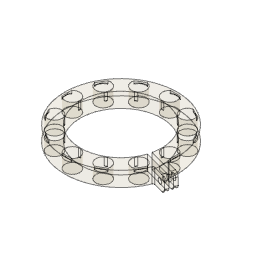
clamp-rev3 v4 (Autodesk Fusion 360 design; units mm, degrees)
Autodesk Fusion 360 part; units mm, degrees
note: some values were not read from the file. Set by a fixed rule: which face or edge a step refers to.
sketch "Sketch1" plane through (0, 0, 9.525) normal (0, 0, 1) x (-1, 0, 0) in component "magnet holder"
  arc A0 (0, -47.625) -> (-95.25, -47.625) centre (-47.625, -47.625) ccw
  line L0 (-95.25, -47.625) -> (-95.25, -130.175)
  arc A1 (-95.25, -130.175) -> (0, -130.175) centre (-47.625, -130.175) ccw
  line L1 (0, -130.175) -> (0, -47.625)
  circle A2 centre (-47.625, -130.175) radius 35.306
  circle A3 centre (-47.625, -130.175) radius 47.625
  circle A4 centre (-47.625, -130.175) radius 35.306
  circle A5 centre (-47.625, -41.275) radius 39.37
  circle A6 centre (-18.3045, -159.4955) radius 2.159
  circle A7 centre (-76.9455, -159.4955) radius 2.159
  circle A8 centre (-18.3045, -100.8545) radius 2.159
  circle A9 centre (-76.9455, -100.8545) radius 2.159
  dimension "d96_1" = 4.318
  dimension "d97_1" = 4.318
  dimension "d98_1" = 4.318
  dimension "d99_1" = 4.318
  constraint concentric A1 A3
  constraint concentric A3 A4
  measures "d96_1" diameter of A6
  measures "d97_1" diameter of A7
  measures "d98_1" diameter of A8
  measures "d99_1" diameter of A9
extrude "Extrude1" add sketch "Sketch1" along normal blind 5.588 contours A1 A3 in component "magnet holder"
sketch "Sketch2" plane through (0, 0, 9.525) normal (0, 0, -1) x (1, 0, 0) in component "magnet holder"
  circle A0 centre (47.625, -130.175) radius 35.306
  circle A1 centre (47.625, -130.175) radius 47.625
  circle A2 centre (47.625, -130.175) radius 41.4655 construction
  circle A3 centre (47.625, -88.7095) radius 6
  circle A4 centre (26.8922, -94.2648) radius 6
  circle A5 centre (11.7148, -109.4422) radius 6
  circle A6 centre (6.1595, -130.175) radius 6
  circle A7 centre (11.7148, -150.9077) radius 6
  circle A8 centre (26.8922, -166.0852) radius 6
  circle A9 centre (47.625, -171.6405) radius 6
  circle A10 centre (68.3577, -166.0852) radius 6
  circle A11 centre (83.5352, -150.9078) radius 6
  circle A12 centre (89.0905, -130.175) radius 6
  circle A13 centre (83.5352, -109.4423) radius 6
  circle A14 centre (68.3578, -94.2648) radius 6
  circle A15 centre (76.9455, -100.8545) radius 2.159
  circle A16 centre (18.3045, -100.8545) radius 2.159
  circle A17 centre (18.3045, -159.4955) radius 2.159
  circle A18 centre (76.9455, -159.4955) radius 2.159
  dimension "d91_1" = 12
  dimension "d93_1" = 360
  constraint concentric A0 A2
  constraint coincident A2 A3.centre
  measures "d91_1" diameter of A3
extrude "Extrude2" cut sketch "Sketch2" against normal blind 4.0005 contours A3 | A4 | A5 | A6 | A7 | A8 | A9 | A10 | A11 | A12 | A13 | A14 in component "magnet holder"
sketch "Sketch1 (2)" plane through (0, 0, 15.875) normal (0, 0, 1) x (-1, 0, 0) in component "magnet spacer"
  circle A0 centre (-76.9455, -100.8545) radius 1.651
  circle A1 centre (-18.3045, -100.8545) radius 1.651
  circle A2 centre (-18.3045, -159.4955) radius 1.651
  circle A3 centre (-76.9455, -159.4955) radius 1.651
  circle A4 centre (-47.625, -130.175) radius 35.306
  circle A5 centre (-47.625, -130.175) radius 47.625
  circle A6 centre (-47.625, -130.175) radius 47.625
  circle A7 centre (-18.3045, -159.4955) radius 1.651
  circle A8 centre (-76.9455, -159.4955) radius 1.651
  circle A9 centre (-76.9455, -100.8545) radius 1.651
  circle A10 centre (-18.3045, -100.8545) radius 1.651
  constraint concentric A4 A6
  constraint concentric A2 A7
  constraint concentric A3 A8
  constraint concentric A0 A9
  constraint concentric A1 A10
sketch "Sketch1 (3)" plane through (0, 0, 16.6622) normal (0, 0, 1) x (-1, 0, 0)
  circle A0 centre (-11.7148, -109.4423) radius 6
  circle A1 centre (-83.5352, -150.9077) radius 6
  circle A2 centre (-11.7148, -150.9078) radius 6
  circle A3 centre (-6.1595, -130.175) radius 6
  circle A4 centre (-89.0905, -130.175) radius 6
  circle A5 centre (-26.8922, -94.2648) radius 6
  circle A6 centre (-68.3577, -94.2648) radius 6
  circle A7 centre (-68.3577, -166.0852) radius 6
  circle A8 centre (-26.8922, -166.0852) radius 6
  circle A9 centre (-47.625, -171.6405) radius 6
  circle A10 centre (-83.5352, -109.4422) radius 6
  circle A11 centre (-47.625, -88.7095) radius 6
  circle A12 centre (-76.9455, -159.4955) radius 2.159
  circle A13 centre (-47.625, -130.175) radius 35.306
  circle A14 centre (-76.9455, -100.8545) radius 2.159
  circle A15 centre (-18.3045, -159.4955) radius 2.159
  circle A16 centre (-18.3045, -100.8545) radius 2.159
  circle A17 centre (-47.625, -130.175) radius 47.625
  line L0 (-53.625, -88.7095) -> (-53.625, -82.8628)
  line L1 (-41.6392, -89.1226) -> (-41.6392, -82.7277)
  line L2 (-73.5539, -97.2648) -> (-76.4772, -92.2015)
  line L3 (-62.9674, -91.6297) -> (-66.1648, -86.0915)
  line L4 (-86.5352, -114.6384) -> (-91.5985, -111.7151)
  line L5 (-80.1845, -104.465) -> (-85.7227, -101.2675)
  line L6 (-89.0905, -136.175) -> (-94.9372, -136.175)
  line L7 (-88.6774, -124.1892) -> (-95.0723, -124.1892)
  line L8 (-80.5352, -156.1039) -> (-85.5985, -159.0272)
  line L9 (-86.1703, -145.5174) -> (-91.7085, -148.7148)
  line L10 (-63.1616, -169.0852) -> (-66.0849, -174.1485)
  line L11 (-73.335, -162.7345) -> (-76.5325, -168.2727)
  line L12 (-41.625, -171.6405) -> (-41.625, -177.4872)
  line L13 (-53.6108, -171.2274) -> (-53.6108, -177.6223)
  line L14 (-21.6961, -163.0852) -> (-18.7728, -168.1485)
  line L15 (-32.2826, -168.7203) -> (-29.0852, -174.2585)
  line L16 (-8.7148, -145.7116) -> (-3.6515, -148.6349)
  line L17 (-15.0655, -155.885) -> (-9.5273, -159.0825)
  line L18 (-6.1595, -124.175) -> (-0.3128, -124.175)
  line L19 (-6.5726, -136.1608) -> (-0.1777, -136.1608)
  line L20 (-14.7148, -104.2461) -> (-9.6515, -101.3228)
  line L21 (-9.0797, -114.8326) -> (-3.5415, -111.6352)
  line L22 (-32.0884, -91.2648) -> (-29.1651, -86.2015)
  line L23 (-21.915, -97.6155) -> (-18.7175, -92.0773)
  point P0 (-53.625, -88.7095)
  dimension "d2" = 360
  constraint coincident P0 L0.start
  constraint vertical L0
  constraint coincident A11 L1.start
  constraint vertical L1
sketch "Sketch2 (2)" plane through (0, 0, 16.6622) normal (0, 0, 1) x (-1, 0, 0)
  circle A0 centre (-76.9455, -159.4955) radius 2.159
  circle A1 centre (-47.625, -130.175) radius 35.306
  circle A2 centre (-76.9455, -100.8545) radius 2.159
  circle A3 centre (-18.3045, -159.4955) radius 2.159
  circle A4 centre (-18.3045, -100.8545) radius 2.159
  circle A5 centre (-47.625, -130.175) radius 47.625
  circle A6 centre (-47.625, -130.175) radius 35.306
  circle A7 centre (-11.7148, -109.4423) radius 6
  circle A8 centre (-83.5352, -150.9077) radius 6
  circle A9 centre (-11.7148, -150.9078) radius 6
  circle A10 centre (-6.1595, -130.175) radius 6
  circle A11 centre (-89.0905, -130.175) radius 6
  circle A12 centre (-26.8922, -94.2648) radius 6
  circle A13 centre (-68.3577, -94.2648) radius 6
  circle A14 centre (-68.3577, -166.0852) radius 6
  circle A15 centre (-26.8922, -166.0852) radius 6
  circle A16 centre (-47.625, -171.6405) radius 6
  circle A17 centre (-83.5352, -109.4422) radius 6
  circle A18 centre (-47.625, -88.7095) radius 6
  circle A19 centre (-47.625, -130.175) radius 47.625
  dimension "d61" = 70.612
  constraint concentric A5 A6
  measures "d61" diameter of A6
extrude "Extrude4" add sketch "Sketch2 (2)" along normal blind 7.112 contours A5 A19 | A7 | A8 | A9 | A10 | A11 | A12 | A13 | A14 | A15 | A16 | A17 | A18 sketch seen with x (-1, 0, 0) y (0, 1, 0) z (0, 0, -1) at (95.25, 0, 26.1872) in component "magnet holder"
extrude "Extrude5" cut 12 faces at (66.4689, 94.5562, 9.525) (49.4935, 89.8687, 9.525) (25.3169, 97.0824, 9.525) (10.5654, 105.7158, 9.525) (6.8902, 133.2158, 9.525) (10.9841, 149.046, 9.525) (26.1616, 167.9469, 9.525) (50.8883, 170.7727, 9.525) (67.6271, 167.9469, 9.525) (80.2719, 151.7755, 9.525) (85.5579, 131.1725, 9.525) (81.9599, 112.2599, 9.525) along direction (0, 0, -1) through all in component "magnet holder"
extrude "Extrude6" cut 12 faces at (81.9802, 105.2788, 13.5255) (89.6447, 133.5821, 13.5255) (80.8432, 151.7755, 13.5255) (67.6271, 167.9469, 13.5255) (50.8883, 170.7727, 13.5255) (26.1616, 167.9469, 13.5255) (10.9841, 149.046, 13.5255) (6.6045, 131.9486, 13.5255) (10.1395, 112.2599, 13.5255) (28.8699, 95.1458, 13.5255) (49.4935, 89.8687, 13.5255) (67.3578, 90.2795, 13.5255) along direction (0, 0, 1) blind 0.5842 in component "magnet holder"
sketch "Sketch3" plane through (0, 0, 23.7742) normal (0, 0, 1) x (-1, 0, 0)
  circle A0 centre (-6.1595, -130.175) radius 6
  circle A1 centre (-26.8922, -166.0852) radius 6
  circle A2 centre (-68.3577, -166.0852) radius 6
  circle A3 centre (-89.0905, -130.175) radius 6
  circle A4 centre (-68.3577, -94.2648) radius 6
  circle A5 centre (-26.8922, -94.2648) radius 6
  circle A6 centre (-47.625, -88.7095) radius 6
  circle A7 centre (-83.5352, -109.4422) radius 6
  circle A8 centre (-83.5352, -150.9077) radius 6
  circle A9 centre (-47.625, -171.6405) radius 6
  circle A10 centre (-11.7148, -150.9078) radius 6
  circle A11 centre (-11.7148, -109.4423) radius 6
  circle A12 centre (-18.3045, -159.4955) radius 2.159
  circle A13 centre (-18.3045, -100.8545) radius 2.159
  circle A14 centre (-76.9455, -100.8545) radius 2.159
  circle A15 centre (-76.9455, -159.4955) radius 2.159
  circle A16 centre (-47.625, -130.175) radius 35.306
  circle A17 centre (-47.625, -130.175) radius 47.625
  circle A18 centre (-47.625, -130.175) radius 47.875
  dimension "d10" = 0.25
  constraint concentric A16 A18
  measures "d10" distance of A17 A18
extrude "Extrude7" add sketch "Sketch3" against normal up to surface (12.7 mm away) contours A18 sketch seen with x (-1, 0, 0) y (0, 1, 0) z (0, 0, -1) at (95.25, 0, 26.1872) in component "magnet holder"
move_face "OffsetFaces1" offset -0.254 3 faces at (42.0961, 169.3099, 4.7837) (42.0961, 173.9711, 12.192) (42.0961, 173.9711, 13.915) in component "magnet holder"
move_face "OffsetFaces2" offset -0.254 3 faces at (73.8866, 163.7546, 4.7837) (63.0884, 163.2157, 12.192) (63.238, 162.9566, 13.915) in component "magnet holder"
move_face "OffsetFaces3" offset -0.254 3 faces at (89.064, 148.5771, 4.7837) (78.0063, 153.2384, 12.192) (77.897, 152.9599, 13.7202) in component "magnet holder"
move_face "OffsetFaces4" offset -0.254 3 faces at (83.5616, 132.5056, 7.1543) (83.5616, 132.5056, 12.192) (83.4523, 132.2271, 13.7202) in component "magnet holder"
move_face "OffsetFaces5" offset -0.254 3 faces at (89.5054, 108.8448, 4.7837) (77.565, 110.0397, 12.192) (77.5426, 109.7413, 13.7202) in component "magnet holder"
move_face "OffsetFaces6" offset -0.254 3 faces at (74.3279, 93.6674, 4.7837) (62.3876, 94.8622, 12.192) (62.3652, 94.5639, 13.7202) in component "magnet holder"
move_face "OffsetFaces7" offset -0.254 3 faces at (53.5952, 88.1121, 4.7837) (41.6548, 89.3069, 12.192) (41.6325, 89.0086, 13.7202) in component "magnet holder"
move_face "OffsetFaces8" offset -0.254 3 faces at (32.8624, 93.6674, 4.7837) (32.8624, 94.8622, 12.192) (32.8624, 94.8622, 13.7202) in component "magnet holder"
move_face "OffsetFaces9" offset -0.254 3 faces at (17.685, 108.8448, 4.7837) (17.685, 110.0397, 12.192) (17.685, 110.0397, 13.7202) in component "magnet holder"
move_face "OffsetFaces10" offset -0.254 3 faces at (0.6306, 132.5056, 7.1543) (0.6306, 132.5056, 12.192) (0.6306, 132.5056, 13.915) in component "magnet holder"
move_face "OffsetFaces11" offset -0.254 3 faces at (6.186, 148.5771, 4.7837) (6.186, 153.2384, 12.192) (6.186, 153.2384, 13.915) in component "magnet holder"
move_face "OffsetFaces12" offset -0.254 3 faces at (32.4211, 163.7546, 4.7837) (32.012, 162.9566, 12.192) (32.012, 162.9566, 13.915) in component "magnet holder"
sketch "Sketch4" plane through (0, 0, 23.7742) normal (0, 0, 1) x (-1, 0, 0)
  circle A0 centre (-47.625, -130.175) radius 47.875
  circle A1 centre (-18.3045, -159.4955) radius 2.159
  circle A2 centre (-18.3045, -100.8545) radius 2.159
  circle A3 centre (-76.9455, -100.8545) radius 2.159
  circle A4 centre (-76.9455, -159.4955) radius 2.159
  arc A5 (-66.1364, -160.239) -> (-64.4055, -161.2383) centre (-68.3577, -166.0852) ccw
  arc A6 (-77.689, -148.6864) -> (-66.1364, -160.239) centre (-47.625, -130.175) ccw
  arc A7 (-78.6883, -146.9555) -> (-77.689, -148.6864) centre (-83.5352, -150.9077) ccw
  arc A8 (-82.9169, -131.1743) -> (-78.6883, -146.9555) centre (-47.625, -130.175) ccw
  arc A9 (-82.9169, -129.1757) -> (-82.9169, -131.1743) centre (-89.0905, -130.175) ccw
  arc A10 (-78.6883, -113.3945) -> (-82.9169, -129.1757) centre (-47.625, -130.175) ccw
  arc A11 (-77.689, -111.6636) -> (-78.6883, -113.3945) centre (-83.5352, -109.4422) ccw
  arc A12 (-66.1364, -100.111) -> (-77.689, -111.6636) centre (-47.625, -130.175) ccw
  arc A13 (-64.4055, -99.1117) -> (-66.1364, -100.111) centre (-68.3577, -94.2648) ccw
  arc A14 (-48.6243, -94.8831) -> (-64.4055, -99.1117) centre (-47.625, -130.175) ccw
  arc A15 (-46.6257, -94.8831) -> (-48.6243, -94.8831) centre (-47.625, -88.7095) ccw
  arc A16 (-30.8445, -99.1117) -> (-46.6257, -94.8831) centre (-47.625, -130.175) ccw
  arc A17 (-29.1136, -100.111) -> (-30.8445, -99.1117) centre (-26.8922, -94.2648) ccw
  arc A18 (-17.561, -111.6636) -> (-29.1136, -100.111) centre (-47.625, -130.175) ccw
  arc A19 (-16.5617, -113.3945) -> (-17.561, -111.6636) centre (-11.7148, -109.4423) ccw
  arc A20 (-12.3331, -129.1757) -> (-16.5617, -113.3945) centre (-47.625, -130.175) ccw
  arc A21 (-12.3331, -131.1743) -> (-12.3331, -129.1757) centre (-6.1595, -130.175) ccw
  arc A22 (-16.5617, -146.9555) -> (-12.3331, -131.1743) centre (-47.625, -130.175) ccw
  arc A23 (-17.561, -148.6864) -> (-16.5617, -146.9555) centre (-11.7148, -150.9078) ccw
  arc A24 (-29.1136, -160.239) -> (-17.561, -148.6864) centre (-47.625, -130.175) ccw
  arc A25 (-30.8445, -161.2383) -> (-29.1136, -160.239) centre (-26.8922, -166.0852) ccw
  arc A26 (-46.6257, -165.4669) -> (-30.8445, -161.2383) centre (-47.625, -130.175) ccw
  arc A27 (-48.6243, -165.4669) -> (-46.6257, -165.4669) centre (-47.625, -171.6405) ccw
  arc A28 (-64.4055, -161.2383) -> (-48.6243, -165.4669) centre (-47.625, -130.175) ccw
  circle A29 centre (-47.625, -130.175) radius 46.2875
  dimension "d25" = 1.5875
  constraint concentric A0 A29
  measures "d25" distance of A0 A29
extrude "Extrude8" add sketch "Sketch4" against normal blind 1.27 contours A0 | A5 A29 | A7 A29 | A27 A29 | A9 A29 | A25 A29 | A11 A29 | A23 A29 | A13 A29 | A21 A29 | A15 A29 | A19 A29 | A17 A29 sketch seen with x (-1, 0, 0) y (0, 1, 0) z (0, 0, -1) at (95.25, 0, 26.1872) in component "magnet holder"
fillet "Fillet1" radius 1.27 1 edges at (47.625, 177.8945, 3.683) in component "magnet holder"
fillet "Fillet2" radius 1.27 1 edges at (71.4848, 171.5013, 3.683) in component "magnet holder"
fillet "Fillet3" radius 1.27 1 edges at (88.9513, 154.0348, 3.683) in component "magnet holder"
fillet "Fillet4" radius 1.27 1 edges at (95.3445, 130.175, 3.683) in component "magnet holder"
fillet "Fillet5" radius 1.27 1 edges at (88.9513, 106.3153, 3.683) in component "magnet holder"
fillet "Fillet6" radius 1.27 1 edges at (71.4848, 88.8487, 3.683) in component "magnet holder"
fillet "Fillet7" radius 1.27 1 edges at (47.625, 82.4555, 3.683) in component "magnet holder"
fillet "Fillet8" radius 1.27 1 edges at (23.7652, 88.8487, 3.683) in component "magnet holder"
fillet "Fillet9" radius 1.27 1 edges at (6.2987, 106.3152, 3.683) in component "magnet holder"
fillet "Fillet10" radius 1.27 1 edges at (-0.0945, 130.175, 3.683) in component "magnet holder"
fillet "Fillet11" radius 1.27 1 edges at (6.2987, 154.0348, 3.683) in component "magnet holder"
fillet "Fillet12" radius 1.27 1 edges at (23.7652, 171.5013, 3.683) in component "magnet holder"
ref_plane "WorkPlane1" through (47.625, 130.175, 24.5362) normal (0.258819, 0.965926, 0) x (0, 0, -1)
ref_plane "WorkPlane2" through (93.8687, 117.784, 17.4242) normal (0.965926, -0.258819, 0) x (-0.258819, -0.965926, 0)
sketch "Sketch10" plane through (93.8687, 117.784, 17.4242) normal (0.965926, -0.258819, 0) x (-0.258819, -0.965926, 0)
  line L0 (-4.7625, -6.35) -> (4.7625, -6.35)
  line L1 (4.7625, -6.35) -> (4.7625, 6.35)
  line L2 (4.7625, 6.35) -> (-4.7625, 6.35)
  line L3 (-4.7625, 6.35) -> (-4.7625, -6.35)
  line L4 (-4.7625, -6.35) -> (4.7625, 6.35) construction
  line L5 (4.7625, -6.35) -> (-4.7625, 6.35) construction
  line L6 (-1.5875, -6.35) -> (1.5875, -6.35)
  line L7 (1.5875, -6.35) -> (1.5875, 6.35)
  line L8 (1.5875, 6.35) -> (-1.5875, 6.35)
  line L9 (-1.5875, 6.35) -> (-1.5875, -6.35)
  line L10 (-1.5875, -6.35) -> (1.5875, 6.35) construction
  line L11 (1.5875, -6.35) -> (-1.5875, 6.35) construction
  dimension "d44" = 9.525
  dimension "d45" = 3.175
  constraint perpendicular L0 L1
  constraint parallel L0 L2
  constraint parallel L1 L3
  constraint horizontal L0
  constraint coincident L4 origin
  constraint coincident L5 origin
  constraint perpendicular L6 L7
  constraint parallel L6 L8
  constraint parallel L7 L9
  constraint horizontal L6
  constraint coincident L10 origin
  constraint coincident L11 origin
  measures "d44" distance of L1.end L2.end
  measures "d45" distance of L7.end L8.end
extrude "Extrude9" cut sketch "Sketch10" against normal blind 25.4 contours L0 L2 L6 L7 L8 L9 sketch seen with x (-1, 0, 0) y (0, 1, 0) z (0, 0, -1) at (95.25, 0, 26.1872) in component "magnet holder"
extrude "Extrude10" add sketch "Sketch10" along normal blind 12.7 and the other way blind 2.54 contours L0 L2 L3 L9 | L0 L1 L2 L7 sketch seen with x (-1, 0, 0) y (0, 1, 0) z (0, 0, -1) at (95.25, 0, 26.1872) in component "magnet holder"
fillet "Fillet13" radius 3.175 4 edges at (-10.0642, 111.4302, 15.113) (-11.7077, 117.5639, 15.113) (-10.0642, 111.4302, 2.413) (-11.7077, 117.5639, 2.413) in component "magnet holder"
fillet "Fillet14" radius 1.27 2 edges at (2.8433, 113.2453, 8.763) (0.3781, 122.4457, 8.763) in component "magnet holder"
sketch "Sketch11" plane through (34.5014, 128.761, 0) normal (-0.258819, -0.965926, 0) x (0.965926, -0.258819, 0)
  line L0 (61.0838, 23.7742) -> (61.0838, 11.0742)
  line L1 (61.0838, 11.0742) -> (69.7104, 11.0742)
  arc A0 (69.7104, 11.0742) -> (72.8854, 14.2492) centre (69.7104, 14.2492) ccw
  line L2 (72.8854, 14.2492) -> (72.8854, 20.5992)
  arc A1 (72.8854, 20.5992) -> (69.7104, 23.7742) centre (69.7104, 20.5992) ccw
  line L3 (69.7104, 23.7742) -> (61.0838, 23.7742)
  circle A2 centre (67.3292, 17.4242) radius 2.0955
  dimension "d54" = 5.5563
  dimension "d55" = 4.191
  measures "d54" distance of L2 A2.centre
  measures "d55" diameter of A2
extrude "Extrude11" cut sketch "Sketch11" against normal blind 17.78 contours A2 sketch seen with x (-1, 0, 0) y (0, 1, 0) z (0, 0, -1) at (95.25, 0, 26.1872) in component "magnet holder"
sketch "Sketch12" plane through (36.9666, 137.9614, 0) normal (0.258819, 0.965926, 0) x (-0.965926, 0.258819, 0)
  circle A0 centre (-67.3292, 17.4242) radius 2.0955
  line L0 (-61.0838, 11.0742) -> (-61.0838, 23.7742)
  line L1 (-61.0838, 23.7742) -> (-69.7104, 23.7742)
  arc A1 (-69.7104, 23.7742) -> (-72.8854, 20.5992) centre (-69.7104, 20.5992) ccw
  line L2 (-72.8854, 20.5992) -> (-72.8854, 14.2492)
  arc A2 (-72.8854, 14.2492) -> (-69.7104, 11.0742) centre (-69.7104, 14.2492) ccw
  line L3 (-69.7104, 11.0742) -> (-61.0838, 11.0742)
  circle A3 centre (-67.3292, 17.4242) radius 2.667
  dimension "d58" = 5.334
  constraint concentric A0 A3
  measures "d58" diameter of A3
extrude "Extrude12" cut sketch "Sketch12" against normal blind 3.81 contours A3 sketch seen with x (-1, 0, 0) y (0, 1, 0) z (0, 0, -1) at (95.25, 0, 26.1872) in component "magnet holder"
delete_face "DeleteFace1" 2 faces at (16.1481, 159.6032, 7.1543) (16.1562, 159.7105, 11.3877) in component "magnet holder"
delete_face "DeleteFace2" 2 faces at (20.4527, 101.0694, 7.1543) (20.4527, 101.0694, 11.3877) in component "magnet holder"
delete_face "DeleteFace3" 2 faces at (78.9743, 160.234, 4.7837) (74.7973, 159.7105, 11.3877) in component "magnet holder"
delete_face "DeleteFace4" 2 faces at (79.0938, 101.0694, 7.1543) (79.0938, 101.0694, 11.3877) in component "magnet holder"
sketch "Sketch14" plane through (0, 0, 23.7742) normal (0, 0, 1) x (-1, 0, 0)
  line L0 (-103.48, -116.8522) -> (-104.3018, -119.919)
  line L1 (-104.3018, -119.919) -> (-95.9691, -122.1517)
  arc A0 (-95.04, -123.5541) -> (-95.9691, -122.1517) centre (-96.2978, -123.3785) ccw
  arc A1 (-95.04, -123.5541) -> (-91.998, -112.2014) centre (-47.625, -130.175) ccw
  arc A2 (-93.5038, -112.9513) -> (-91.998, -112.2014) centre (-93.1751, -111.7246) ccw
  line L2 (-93.5038, -112.9513) -> (-101.8365, -110.7186)
  line L3 (-101.8365, -110.7186) -> (-102.6583, -113.7854)
  line L4 (-102.6583, -113.7854) -> (-81.2826, -119.513)
  arc A3 (-78.6883, -113.3945) -> (-81.2826, -119.513) centre (-47.625, -130.175) ccw
  arc A4 (-89.6472, -110.7671) -> (-78.6883, -113.3945) centre (-83.5352, -109.4423) ccw
  arc A5 (-85.4438, -103.4866) -> (-89.6472, -110.7671) centre (-47.625, -130.175) ccw
  arc A6 (-77.689, -111.6636) -> (-85.4438, -103.4866) centre (-83.5352, -109.4423) ccw
  arc A7 (-66.1364, -100.111) -> (-77.689, -111.6636) centre (-47.625, -130.175) ccw
  arc A8 (-74.3134, -92.3562) -> (-66.1364, -100.111) centre (-68.3577, -94.2648) ccw
  arc A9 (-67.0329, -88.1528) -> (-74.3134, -92.3562) centre (-47.625, -130.175) ccw
  arc A10 (-64.4055, -99.1117) -> (-67.0329, -88.1528) centre (-68.3577, -94.2648) ccw
  arc A11 (-48.6243, -94.8831) -> (-64.4055, -99.1117) centre (-47.625, -130.175) ccw
  arc A12 (-51.8284, -84.0788) -> (-48.6243, -94.8831) centre (-47.625, -88.7095) ccw
  arc A13 (-43.4216, -84.0788) -> (-51.8284, -84.0788) centre (-47.625, -130.175) ccw
  arc A14 (-46.6257, -94.8831) -> (-43.4216, -84.0788) centre (-47.625, -88.7095) ccw
  arc A15 (-30.8445, -99.1117) -> (-46.6257, -94.8831) centre (-47.625, -130.175) ccw
  arc A16 (-28.2171, -88.1528) -> (-30.8445, -99.1117) centre (-26.8922, -94.2648) ccw
  arc A17 (-20.9366, -92.3562) -> (-28.2171, -88.1528) centre (-47.625, -130.175) ccw
  arc A18 (-29.1136, -100.111) -> (-20.9366, -92.3562) centre (-26.8922, -94.2648) ccw
  arc A19 (-17.561, -111.6636) -> (-29.1136, -100.111) centre (-47.625, -130.175) ccw
  arc A20 (-9.8062, -103.4866) -> (-17.561, -111.6636) centre (-11.7148, -109.4423) ccw
  arc A21 (-5.6028, -110.7671) -> (-9.8062, -103.4866) centre (-47.625, -130.175) ccw
  arc A22 (-16.5617, -113.3945) -> (-5.6028, -110.7671) centre (-11.7148, -109.4423) ccw
  arc A23 (-12.3331, -129.1757) -> (-16.5617, -113.3945) centre (-47.625, -130.175) ccw
  arc A24 (-1.5288, -125.9716) -> (-12.3331, -129.1757) centre (-6.1595, -130.175) ccw
  arc A25 (-1.5288, -134.3784) -> (-1.5288, -125.9716) centre (-47.625, -130.175) ccw
  arc A26 (-12.3331, -131.1743) -> (-1.5288, -134.3784) centre (-6.1595, -130.175) ccw
  arc A27 (-16.5617, -146.9555) -> (-12.3331, -131.1743) centre (-47.625, -130.175) ccw
  arc A28 (-5.6028, -149.5829) -> (-16.5617, -146.9555) centre (-11.7148, -150.9077) ccw
  arc A29 (-9.8062, -156.8634) -> (-5.6028, -149.5829) centre (-47.625, -130.175) ccw
  arc A30 (-17.561, -148.6864) -> (-9.8062, -156.8634) centre (-11.7148, -150.9077) ccw
  arc A31 (-29.1136, -160.239) -> (-17.561, -148.6864) centre (-47.625, -130.175) ccw
  arc A32 (-20.9366, -167.9938) -> (-29.1136, -160.239) centre (-26.8922, -166.0852) ccw
  arc A33 (-28.2171, -172.1972) -> (-20.9366, -167.9938) centre (-47.625, -130.175) ccw
  arc A34 (-30.8445, -161.2383) -> (-28.2171, -172.1972) centre (-26.8922, -166.0852) ccw
  arc A35 (-46.6257, -165.4669) -> (-30.8445, -161.2383) centre (-47.625, -130.175) ccw
  arc A36 (-43.4216, -176.2712) -> (-46.6257, -165.4669) centre (-47.625, -171.6405) ccw
  arc A37 (-51.8284, -176.2712) -> (-43.4216, -176.2712) centre (-47.625, -130.175) ccw
  arc A38 (-48.6243, -165.4669) -> (-51.8284, -176.2712) centre (-47.625, -171.6405) ccw
  arc A39 (-64.4055, -161.2383) -> (-48.6243, -165.4669) centre (-47.625, -130.175) ccw
  arc A40 (-67.0329, -172.1972) -> (-64.4055, -161.2383) centre (-68.3577, -166.0852) ccw
  arc A41 (-74.3134, -167.9938) -> (-67.0329, -172.1972) centre (-47.625, -130.175) ccw
  arc A42 (-66.1364, -160.239) -> (-74.3134, -167.9938) centre (-68.3577, -166.0852) ccw
  arc A43 (-77.689, -148.6864) -> (-66.1364, -160.239) centre (-47.625, -130.175) ccw
  arc A44 (-85.4438, -156.8634) -> (-77.689, -148.6864) centre (-83.5352, -150.9077) ccw
  arc A45 (-89.6472, -149.5829) -> (-85.4438, -156.8634) centre (-47.625, -130.175) ccw
  arc A46 (-78.6883, -146.9555) -> (-89.6472, -149.5829) centre (-83.5352, -150.9077) ccw
  arc A47 (-82.9169, -131.1743) -> (-78.6883, -146.9555) centre (-47.625, -130.175) ccw
  arc A48 (-93.7212, -134.3784) -> (-82.9169, -131.1743) centre (-89.0905, -130.175) ccw
  arc A49 (-93.7212, -125.9716) -> (-93.7212, -134.3784) centre (-47.625, -130.175) ccw
  arc A50 (-82.9169, -129.1757) -> (-93.7212, -125.9716) centre (-89.0905, -130.175) ccw
  arc A51 (-82.1044, -122.5798) -> (-82.9169, -129.1757) centre (-47.625, -130.175) ccw
  line L5 (-82.1044, -122.5798) -> (-103.48, -116.8522)
  circle A52 centre (-47.625, -130.175) radius 35.306
  circle A53 centre (-47.625, -130.175) radius 34.706
  line L6 (-81.2826, -119.513) -> (-80.7025, -119.6684)
  line L7 (-82.1044, -122.5798) -> (-81.5242, -122.7352)
  dimension "d65" = 0.6
  constraint concentric A1 A52
  constraint coincident L4.end A52
  constraint concentric A1 A53
  constraint coincident L4.end A3.end
  constraint coincident A53 L6.end
  constraint parallel L5 L6
  constraint coincident A51.start L5.start
  constraint coincident A53 L7.end
  constraint parallel L6 L7
  measures "d65" distance of A52 A53
extrude "Extrude15" add sketch "Sketch14" against normal up to surface (12.7 mm away) contours A3 A7 A11 A15 A19 A23 A27 A31 A35 A39 A43 A47 A51 A52 A53 L6 L7 sketch seen with x (-1, 0, 0) y (0, 1, 0) z (0, 0, -1) at (95.25, 0, 26.1872) in component "magnet holder"
sketch "Sketch15" plane through (0, 0, 23.7742) normal (0, 0, 1) x (-1, 0, 0)
sketch "Sketch17" plane through (0, 0, 12.0775) normal (0, 0, 1) x (-1, 0, 0)
  arc A0 (-16.5617, -113.3945) -> (-17.561, -111.6636) centre (-47.625, -130.175) ccw
  arc A1 (-16.5617, -113.3945) -> (-17.561, -111.6636) centre (-11.7148, -109.4423) ccw
  line L0 (-47.625, -130.175) -> (20, -130.175) construction
  circle A2 centre (-11.7148, -109.4423) radius 6.254
  circle A3 centre (-26.8923, -94.2648) radius 6.254
  circle A4 centre (-47.625, -88.7095) radius 6.254
  circle A5 centre (-68.3578, -94.2648) radius 6.254
  circle A6 centre (-83.5352, -109.4423) radius 6.254
  circle A7 centre (-89.0905, -130.175) radius 6.254
  circle A8 centre (-83.5352, -150.9078) radius 6.254
  circle A9 centre (-68.3578, -166.0852) radius 6.254
  circle A10 centre (-47.625, -171.6405) radius 6.254
  circle A11 centre (-26.8923, -166.0852) radius 6.254
  circle A12 centre (-11.7148, -150.9078) radius 6.254
  circle A13 centre (-6.1595, -130.175) radius 6.254
  dimension "d71" = 360
  constraint coincident A0.centre L0.start
  constraint horizontal L0
  constraint concentric A1 A2
extrude "Extrude16" cut sketch "Sketch17" along normal blind 5 contours A0 A1 A2 | A3 | A4 | A5 | A6 | A7 | A8 | A9 | A10 | A11 | A12 | A13 sketch seen with x (-1, 0, 0) y (0, 1, 0) z (0, 0, -1) at (95.25, 0, 26.1872) in component "magnet holder"
sketch "Sketch18" plane through (0, 0, 12.0775) normal (0, 0, 1) x (-1, 0, 0)
  arc A0 (-16.5617, -113.3945) -> (-17.561, -111.6636) centre (-47.625, -130.175) ccw
  arc A1 (-16.5617, -113.3945) -> (-17.561, -111.6636) centre (-11.7148, -109.4423) ccw
  circle A2 centre (-11.7148, -109.4423) radius 6.254
  constraint concentric A1 A2
extrude "Extrude17" cut sketch "Sketch18" along normal blind 5 contours A0 A2 sketch seen with x (-1, 0, 0) y (0, 1, 0) z (0, 0, -1) at (95.25, 0, 26.1872) in component "magnet holder"
component "magnet holder" placed x (-1, 0, 0) y (0, 1, 0) z (0, 0, -1) at (95.25, 0, 26.1872)
component "magnet spacer" placed x (1, 0, 0) y (0, 1, 0) z (0, 0, 1) at (0, 104.14, -5.5626)
equation "d91_1 = ( 12 / 25.4 ) * 1 in"
equation "d94_1 = ( -3 / 16 ) * 1 in + 0.03 in"
equation "d100_1 = 0.22 in"
equation "d101_1 = 0.0 deg"
equation "d5 = 0.5 in - 0.22 in"
equation "d54 = ( 7 / 32 ) * 1 in"
